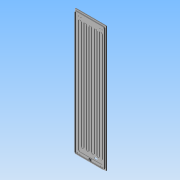
# Autodesk Inventor part: Ply back
Saved by Autodesk Inventor 2013 (Build 170138000, 138)
## iProperties
Created: 2018-07-07
Part Number: Ply back
Material: Generic
Document SubType Name: Modeling
Designer: Jeff Vyduna
Density: 1 g/cm^3
Author: Jeff Vyduna
Autodesk Inventor part; units mm, degrees
ref_plane "YZ Plane" through (0, 0, 0) normal (1, 0, 0) x (0, 1, 0)
ref_plane "XZ Plane" through (0, 0, 0) normal (0, 1, 0) x (-1, 0, 0)
ref_plane "XY Plane" through (0, 0, 0) normal (0, 0, 1) x (1, 0, 0)
sketch "TwoLineColumn" plane through (0, 0, 0) normal (0, 0, 1) x (1, 0, 0)
  line L0 (50.8, -1261.9609) -> (50.8, 922.4391) construction
  line L1 (101.6, -1261.9609) -> (101.6, 922.4391) construction
  arc A0 (101.6, 922.4391) -> (50.8, 922.4391) centre (76.2, 922.4391) ccw construction
  arc A1 (101.6, -1261.9609) -> (152.4, -1261.9609) centre (127, -1261.9609) ccw construction
  line L2 (56.896, -1261.9609) -> (56.896, 922.4391)
  arc A2 (95.504, 922.4391) -> (56.896, 922.4391) centre (76.2, 922.4391) ccw
  line L3 (95.504, 922.4391) -> (95.504, -1261.9609)
  arc A3 (95.504, -1261.9609) -> (158.496, -1261.9609) centre (127, -1261.9609) ccw
  line L4 (44.704, -1261.9609) -> (44.704, 922.4391)
  arc A4 (107.696, 922.4391) -> (44.704, 922.4391) centre (76.2, 922.4391) ccw
  line L5 (107.696, 922.4391) -> (107.696, -1261.9609)
  arc A5 (107.696, -1261.9609) -> (146.304, -1261.9609) centre (127, -1261.9609) ccw
  line L6 (50.8, -1261.9609) -> (152.4, -1261.9609) construction
  dimension "d4" = 2184.4
  dimension "lineSpacing" = 50.8
  dimension "d6" = 25.4
  dimension "d9" = 6.096
  dimension "d10" = 6.096
  measures "d4" distance of L0.start L0.end
  measures "lineSpacing" distance between parallel lines of L1 L0
  measures "d6" radius of A1
  measures "d9" distance between parallel lines of L1 L3
  measures "d10" distance between parallel lines of L5 L1
sketch "TwoLineColumnEnd" plane through (0, 0, 0) normal (0, 0, 1) x (1, 0, 0)
  line L0 (103.0524, -1453.1843) -> (103.0524, 731.2157)
  arc A0 (166.0444, 731.2157) -> (103.0524, 731.2157) centre (134.5484, 731.2157) ccw
  line L1 (166.0444, 731.2157) -> (166.0444, -1453.1843)
  line L2 (109.1484, -1453.1843) -> (109.1484, 731.2157) construction
  line L3 (159.9484, -1453.1843) -> (159.9484, 731.2157) construction
  arc A1 (159.9484, 731.2157) -> (109.1484, 731.2157) centre (134.5484, 731.2157) ccw construction
  line L4 (115.2444, -1453.1843) -> (115.2444, 731.2157)
  arc A2 (153.8524, 731.2157) -> (115.2444, 731.2157) centre (134.5484, 731.2157) ccw
  line L5 (153.8524, 731.2157) -> (153.8524, -1453.1843)
  line L6 (109.1484, -1453.1843) -> (159.9484, -1453.1843) construction
  dimension "d22" = 2184.4
  dimension "d23" = 50.8
  dimension "d25" = 6.096
  dimension "d26" = 6.096
  dimension "d29" = 50.8
  measures "d22" distance of L2.start L2.end
  measures "d23" distance between parallel lines of L3 L2
  measures "d25" distance between parallel lines of L3 L5
  measures "d26" distance between parallel lines of L1 L3
  measures "d29" distance of L2.start L6.end
sketch "15mm Neon profile" plane through (0, 0, 0) normal (0, 0, 1) x (1, 0, 0)
  circle A0 centre (522.6685, 24.7098) radius 6.985 construction
  line L0 (516.6995, 21.082) -> (528.6375, 21.082) construction
  line L1 (528.6375, 21.082) -> (528.6375, 6.35) construction
  line L2 (528.6375, 6.35) -> (516.6995, 6.35) construction
  line L3 (516.6995, 6.35) -> (516.6995, 21.082) construction
  point P0 (522.6685, 16.011)
  dimension "d73" = 13.97
  dimension "d74" = 11.938
  dimension "d76" = 14.732
  measures "d73" diameter of A0
  measures "d74" distance of L0.start L0.end
  measures "d76" distance of L0.end L1.end
sketch "U Bolt hole and bore" plane through (0, 0, 0) normal (0, 0, 1) x (1, 0, 0)
  circle A0 centre (40.0435, 30.4025) radius 9.525
  circle A1 centre (74.9685, 30.4025) radius 9.525
  circle A2 centre (40.0435, 30.4025) radius 3.9688
  circle A3 centre (74.9685, 30.4025) radius 3.9688
  point P0 (68.2625, 33.02)
  dimension "d100" = 19.05
  dimension "d102" = 34.925
  dimension "d105" = 7.9375
  measures "d100" diameter of A0
  measures "d102" distance of A1.centre A0.centre
  measures "d105" diameter of A2
sketch "Stock" plane through (0, 0, 0) normal (0, 0, 1) x (1, 0, 0)
  line L0 (0, 0) -> (604.8375, 0)
  line L1 (604.8375, 0) -> (604.8375, 2438.4)
  line L2 (604.8375, 2438.4) -> (0, 2438.4)
  line L3 (0, 2438.4) -> (0, 0)
  dimension "d1" = 604.8375
  dimension "d2" = 2438.4
  constraints: 8 end point, 2 parallel, 1 coincident, 1 horizontal, 1 perpendicular
  measures "d1" distance of L2.end L1.end
  measures "d2" distance of L1.end L0.end
extrude "Stock Extrusion" add sketch "Stock" along normal blind 19.05
sketch "LEDPocket" plane through (0, 0, 19.05) normal (0, 0, 1) x (1, 0, 0)
  line L0 (0, 0) -> (604.8375, 0)
  line L1 (604.8375, 0) -> (604.8375, 2438.4)
  line L2 (63.5, 2438.4) -> (63.5, 0) construction
  line L3 (541.3375, 2438.4) -> (541.3375, 0) construction
  line L4 (474.1228, 177.8) -> (474.1228, 2266.95)
  arc A0 (537.1148, 2266.95) -> (474.1228, 2266.95) centre (505.6188, 2266.95) ccw
  line L5 (537.1148, 2266.95) -> (537.1148, 88.9)
  line L6 (480.2188, 177.8) -> (480.2188, 2266.95) construction
  line L7 (531.0188, 177.8) -> (531.0188, 2266.95) construction
  arc A1 (531.0188, 2266.95) -> (480.2188, 2266.95) centre (505.6188, 2266.95) ccw construction
  line L8 (486.3148, 177.8) -> (486.3148, 2266.95)
  arc A2 (524.9228, 2266.95) -> (486.3148, 2266.95) centre (505.6188, 2266.95) ccw
  line L9 (524.9228, 2266.95) -> (524.9228, 152.4)
  line L10 (67.7227, 88.9) -> (67.7227, 2266.95)
  arc A3 (130.7147, 2266.95) -> (67.7227, 2266.95) centre (99.2187, 2266.95) ccw
  line L11 (130.7147, 2266.95) -> (130.7147, 177.8)
  arc A4 (130.7147, 177.8) -> (169.3227, 177.8) centre (150.0187, 177.8) ccw
  line L12 (73.8187, 177.8) -> (73.8187, 2266.95) construction
  line L13 (124.6187, 177.8) -> (124.6187, 2266.95) construction
  arc A5 (124.6187, 2266.95) -> (73.8187, 2266.95) centre (99.2187, 2266.95) ccw construction
  arc A6 (124.6187, 177.8) -> (175.4187, 177.8) centre (150.0187, 177.8) ccw construction
  line L14 (79.9147, 152.4) -> (79.9147, 2266.95)
  arc A7 (118.5227, 2266.95) -> (79.9147, 2266.95) centre (99.2187, 2266.95) ccw
  line L15 (118.5227, 2266.95) -> (118.5227, 177.8)
  arc A8 (118.5227, 177.8) -> (181.5147, 177.8) centre (150.0187, 177.8) ccw
  line L16 (169.3227, 177.8) -> (169.3227, 2266.95)
  arc A9 (232.3147, 2266.95) -> (169.3227, 2266.95) centre (200.8187, 2266.95) ccw
  line L17 (232.3147, 2266.95) -> (232.3147, 177.8)
  arc A10 (232.3147, 177.8) -> (270.9227, 177.8) centre (251.6187, 177.8) ccw
  line L18 (175.4187, 177.8) -> (175.4187, 2266.95) construction
  line L19 (226.2187, 177.8) -> (226.2187, 2266.95) construction
  arc A11 (226.2187, 2266.95) -> (175.4187, 2266.95) centre (200.8187, 2266.95) ccw construction
  arc A12 (226.2187, 177.8) -> (277.0187, 177.8) centre (251.6187, 177.8) ccw construction
  line L20 (181.5147, 177.8) -> (181.5147, 2266.95)
  arc A13 (220.1227, 2266.95) -> (181.5147, 2266.95) centre (200.8187, 2266.95) ccw
  line L21 (220.1227, 2266.95) -> (220.1227, 177.8)
  arc A14 (220.1227, 177.8) -> (283.1148, 177.8) centre (251.6187, 177.8) ccw
  line L22 (270.9227, 177.8) -> (270.9227, 2266.95)
  arc A15 (333.9147, 2266.95) -> (270.9227, 2266.95) centre (302.4187, 2266.95) ccw
  line L23 (333.9147, 2266.95) -> (333.9148, 177.8)
  arc A16 (333.9148, 177.8) -> (372.5227, 177.8) centre (353.2187, 177.8) ccw
  line L24 (277.0187, 177.8) -> (277.0187, 2266.95) construction
  line L25 (327.8187, 177.8) -> (327.8187, 2266.95) construction
  arc A17 (327.8187, 2266.95) -> (277.0187, 2266.95) centre (302.4187, 2266.95) ccw construction
  arc A18 (327.8187, 177.8) -> (378.6188, 177.8) centre (353.2187, 177.8) ccw construction
  line L26 (283.1148, 177.8) -> (283.1148, 2266.95)
  arc A19 (321.7227, 2266.95) -> (283.1148, 2266.95) centre (302.4187, 2266.95) ccw
  line L27 (321.7227, 2266.95) -> (321.7227, 177.8)
  arc A20 (321.7227, 177.8) -> (384.7148, 177.8) centre (353.2187, 177.8) ccw
  line L28 (372.5227, 177.8) -> (372.5227, 2266.95)
  arc A21 (435.5148, 2266.95) -> (372.5227, 2266.95) centre (404.0188, 2266.95) ccw
  line L29 (435.5148, 2266.95) -> (435.5148, 177.8)
  arc A22 (435.5148, 177.8) -> (474.1228, 177.8) centre (454.8188, 177.8) ccw
  line L30 (378.6188, 177.8) -> (378.6188, 2266.95) construction
  line L31 (429.4188, 177.8) -> (429.4188, 2266.95) construction
  arc A23 (429.4188, 2266.95) -> (378.6188, 2266.95) centre (404.0188, 2266.95) ccw construction
  arc A24 (429.4188, 177.8) -> (480.2188, 177.8) centre (454.8188, 177.8) ccw construction
  line L32 (384.7148, 177.8) -> (384.7148, 2266.95)
  arc A25 (423.3227, 2266.95) -> (384.7148, 2266.95) centre (404.0188, 2266.95) ccw
  line L33 (423.3227, 2266.95) -> (423.3227, 177.8)
  arc A26 (423.3227, 177.8) -> (486.3148, 177.8) centre (454.8188, 177.8) ccw
  line L34 (499.5228, 127) -> (105.3147, 127)
  line L35 (63.5, 2374.9) -> (541.3375, 2374.9) construction
  arc A27 (79.9147, 152.4) -> (105.3147, 127) centre (105.3147, 152.4) ccw
  arc A28 (67.7227, 88.9) -> (93.1227, 63.5) centre (93.1227, 88.9) ccw
  arc A29 (499.5228, 127) -> (524.9228, 152.4) centre (499.5228, 152.4) ccw
  arc A30 (511.7148, 63.5) -> (537.1148, 88.9) centre (511.7148, 88.9) ccw
  line L36 (93.1227, 63.5) -> (511.7148, 63.5)
  line L37 (0, 2438.4) -> (0, 0) projected
  line L38 (604.8375, 2438.4) -> (0, 2438.4) projected
  line L39 (63.5, 2311.4) -> (541.3375, 2311.4) construction
  point P0 (79.9147, 127)
  point P1 (524.9228, 127)
  dimension "d21" = 541.3375
  dimension "d42" = 50.8
  dimension "d43" = 6.096
  dimension "d44" = 6.096
  dimension "d50" = 50.8
  dimension "d51" = 25.4
  dimension "d52" = 6.096
  dimension "d53" = 6.096
  dimension "d202" = 50.8
  dimension "d204" = 25.4
  dimension "d205" = 63.5
  dimension "d206" = 63.5
  dimension "d208" = 302.4187
  dimension "d209" = 63.5
  dimension "d210" = 63.5
  dimension "d211" = 25.4
  dimension "d212" = 44.45
  dimension "d213" = 63.5
  constraints: 76 end point, 62 point on circle, 60 tangent, 31 centre point, 27 vertical, 12 point on line, 9 horizontal alignment, 8 equal radius, 2 horizontal, 1 perpendicular
  measures "d21" distance from line of L0.start L3
  measures "d42" distance between parallel lines of L7 L6
  measures "d43" distance between parallel lines of L7 L9
  measures "d44" distance between parallel lines of L5 L7
  measures "d50" distance between parallel lines of L13 L12
  measures "d51" radius of A6
  measures "d52" distance between parallel lines of L13 L15
  measures "d53" distance between parallel lines of L11 L13
  measures "d202" distance from line of L34 A4.centre
  measures "d204" radius of A27
  measures "d205" distance between parallel lines of L36 L34
  measures "d206" distance between parallel lines of L0 L36
  measures "d208" distance from line of L37 A15.centre
  measures "d209" distance from line of L35.start L38
  measures "d210" distance of L39.start L35.start
  measures "d211" radius of A28
  measures "d212" vertical distance of A3.centre L39.start
  measures "d213" distance from line of L0.start L2
extrude "Main rope pocket" cut sketch "LEDPocket" against normal blind 12.7 contours L4 A0 L5 A30 L36 A28 L10 A3 L11 A4 L16 A9 L17 A10 L22 A15 L23 A16 L28 A21 L29 A22
sketch "Side profile reference" plane through (0, 0, 0) normal (0, -1, 0) x (1, 0, 0)
  line L0 (0, 0) -> (604.8375, 0) projected
  line L1 (604.8375, 0) -> (604.8375, 19.05) projected
  line L2 (0, 19.05) -> (604.8375, 19.05) projected
  line L3 (0, 0) -> (0, 19.05) projected
  line L4 (598.4875, 38.1) -> (586.2955, 38.1) construction
  line L5 (586.2955, 38.1) -> (586.2955, 25.4) construction
  line L6 (586.2955, 25.4) -> (598.4875, 25.4) construction
  line L7 (598.4875, 25.4) -> (598.4875, 38.1) construction
  line L8 (604.8375, 19.05) -> (541.3375, 19.05) construction
  line L9 (541.3375, 19.05) -> (541.3375, 38.1) construction
  line L10 (541.3375, 38.1) -> (604.8375, 38.1) construction
  line L11 (604.8375, 38.1) -> (604.8375, 19.05) construction
  line L12 (547.6875, 38.1) -> (573.0875, 38.1) construction
  line L13 (573.0875, 38.1) -> (573.0875, 40.64) construction
  line L14 (573.0875, 40.64) -> (547.6875, 40.64) construction
  line L15 (547.6875, 40.64) -> (547.6875, 38.1) construction
  line L16 (579.4375, 40.64) -> (516.6995, 40.64) construction
  line L17 (516.6995, 40.64) -> (516.6995, 45.847) construction
  line L18 (516.6995, 45.847) -> (579.4375, 45.847) construction
  line L19 (579.4375, 45.847) -> (579.4375, 40.64) construction
  circle A0 centre (522.6685, 24.7098) radius 6.985 construction
  line L20 (516.6995, 21.082) -> (528.6375, 21.082) construction
  line L21 (528.6375, 21.082) -> (528.6375, 6.35) construction
  line L22 (528.6375, 6.35) -> (516.6995, 6.35) construction
  line L23 (516.6995, 6.35) -> (516.6995, 21.082) construction
  circle A1 centre (592.3915, 43.7598) radius 6.985 construction
  line L24 (586.4225, 40.132) -> (598.3605, 40.132) construction
  line L25 (598.3605, 40.132) -> (598.3605, 25.4) construction
  line L26 (598.3605, 25.4) -> (586.4225, 25.4) construction
  line L27 (586.4225, 25.4) -> (586.4225, 40.132) construction
  point P0 (566.7375, 19.05)
  point P1 (592.3915, 25.4)
  point P2 (592.3915, 25.4)
  dimension "d75" = 12.7
  dimension "d80" = 12.192
  dimension "d88" = 6.35
  dimension "d90" = 63.5
  dimension "d91" = 19.05
  dimension "d92" = 25.4
  dimension "d93" = 2.54
  dimension "d94" = 6.35
  dimension "d95" = 12.7
  dimension "d96" = 6.35
  dimension "d97" = 5.207
  dimension "d98" = 0
  dimension "d99" = 12.7
  constraints: 32 end point, 8 parallel, 5 horizontal, 4 perpendicular, 1 coincident, 1 collinear, 1 midpoint, 1 point on line, 1 other
  measures "d80" distance of L6.end L5.end
  measures "d88" horizontal distance of L1.end L6.end
  measures "d90" distance of L9.end L10.end
  measures "d91" distance of L8.end L9.end
  measures "d92" distance of L14.end L13.end
  measures "d93" distance of L13.end L12.end
  measures "d94" distance of L9.end L12.start
  measures "d96" horizontal distance of L16.start L12.end
  measures "d97" distance of L16.end L17.end
  measures "d99" vertical distance of L10.end L6.end
sketch "U-Bolt holes" plane through (0, 0, 19.05) normal (0, 0, 1) x (1, 0, 0)
  line L0 (0, 0) -> (604.8375, 0) projected
  line L1 (604.8375, 0) -> (604.8375, 2438.4) projected
  line L2 (0, 2438.4) -> (0, 0) projected
  line L3 (604.8375, 2438.4) -> (0, 2438.4) projected
  point P0 (53.975, 33.02)
  point P1 (100.0125, 33.02)
  point P2 (504.825, 33.02)
  point P3 (550.8625, 33.02)
  point P4 (531.8125, 2344.42)
  point P5 (485.775, 2344.42)
  point P6 (73.025, 2344.42)
  point P7 (119.0625, 2344.42)
  dimension "d109" = 33.02
  dimension "uBoltSpacing" = 46.0375
  dimension "d111" = 46.0375
  dimension "d112" = 19.05
  dimension "d113" = 53.975
  dimension "d114" = 53.975
  dimension "d115" = 46.0375
  dimension "d116" = 46.0375
  dimension "d117" = 19.05
  dimension "d126" = 93.98
  dimension "d198" = 2311.4
  constraints: 6 horizontal alignment
  measures "d109" distance from line of L0 point (53.975, 33.02)
  measures "uBoltSpacing" distance of point (100.012, 33.02) point (53.975, 33.02)
  measures "d111" distance of point (550.862, 33.02) point (504.825, 33.02)
  measures "d112" horizontal distance of point (53.975, 33.02) point (73.025, 2344.42)
  measures "d113" distance from line of L1 point (550.862, 33.02)
  measures "d114" distance from line of L2 point (53.975, 33.02)
  measures "d115" distance of point (73.025, 2344.42) point (119.062, 2344.42)
  measures "d116" distance of point (531.812, 2344.42) point (485.775, 2344.42)
  measures "d117" horizontal distance of point (531.812, 2344.42) point (550.862, 33.02)
  measures "d126" distance from line of L3 point (73.025, 2344.42)
  measures "d198" vertical distance of point (73.025, 2344.42) point (53.975, 33.02)
hole "Hole1" at (73.025, 2344.42, 19.05) at (119.0625, 2344.42, 19.05) at (485.775, 2344.42, 19.05) at (531.8125, 2344.42, 19.05) at (550.8625, 33.02, 19.05) at (504.825, 33.02, 19.05) at (100.0125, 33.02, 19.05) at (53.975, 33.02, 19.05) direction (0, 0, -1) diameter 7.9375 end through all counterbore diameter 19.05 counterbore depth 6.35
ref_plane "Work Plane1" through (0, 0, 6.35) normal (0, 0, 1) x (1, 0, 0)
sketch "WeatherProof panel" plane through (0, 0, 6.35) normal (0, 0, 1) x (1, 0, 0)
  line L0 (370.9353, 127) -> (418.5603, 127)
  line L1 (423.3228, 122.2375) -> (423.3228, 87.3125)
  line L2 (418.5603, 82.55) -> (370.9353, 82.55)
  line L3 (366.1728, 87.3125) -> (366.1728, 122.2375)
  arc A0 (370.9353, 127) -> (366.1728, 122.2375) centre (370.9353, 122.2375) ccw
  arc A1 (366.1728, 87.3125) -> (370.9353, 82.55) centre (370.9353, 87.3125) ccw
  arc A2 (423.3228, 122.2375) -> (418.5603, 127) centre (418.5603, 122.2375) ccw
  arc A3 (418.5603, 82.55) -> (423.3228, 87.3125) centre (418.5603, 87.3125) ccw
  line L4 (105.3147, 127) -> (499.5228, 127) projected
  line L5 (524.9228, 152.4) -> (524.9228, 2266.95) projected
  point P0 (0, 0)
  point P1 (423.3228, 82.55)
  point P2 (423.3228, 127)
  point P3 (366.1728, 82.55)
  dimension "d127" = 44.45
  dimension "d129" = 57.15
  dimension "d130" = 4.7625
  dimension "d214" = 101.6
  constraints: 8 end point, 8 point on circle, 8 tangent, 6 point on line, 4 centre point, 3 equal radius, 2 parallel, 1 collinear, 1 horizontal, 1 perpendicular
  measures "d127" distance of point (423.323, 127) point (423.323, 82.55)
  measures "d129" distance of point (423.323, 82.55) point (366.173, 82.55)
  measures "d130" radius of A0
  measures "d214" distance between parallel lines of L5 L1
extrude "Through Panel Extrusion5" cut sketch "WeatherProof panel" against normal through all
sketch "Border" plane through (0, 0, 19.05) normal (0, 0, 1) x (1, 0, 0)
  line L0 (38.989, 2418.461) -> (565.8485, 2418.461) construction
  line L1 (584.8985, 2399.411) -> (584.8985, 38.989) construction
  line L2 (19.939, 38.989) -> (19.939, 2399.411) construction
  line L3 (0, 2438.4) -> (0, 0) construction
  line L4 (604.8375, 2438.4) -> (0, 2438.4) construction
  line L5 (0, 0) -> (604.8375, 0) construction
  arc A0 (19.939, 38.989) -> (38.989, 19.939) centre (38.989, 38.989) ccw construction
  arc A1 (565.8485, 19.939) -> (584.8985, 38.989) centre (565.8485, 38.989) ccw construction
  arc A2 (584.8985, 2399.411) -> (565.8485, 2418.461) centre (565.8485, 2399.411) ccw construction
  arc A3 (38.989, 2418.461) -> (19.939, 2399.411) centre (38.989, 2399.411) ccw construction
  line L6 (511.7148, 63.5) -> (93.1227, 63.5) construction
  line L7 (315.1187, 63.5) -> (315.1187, 38.989) construction
  line L8 (289.7187, 38.989) -> (289.7187, 63.5) construction
  line L9 (565.8485, 19.939) -> (334.1687, 19.939) construction
  line L10 (270.6687, 19.939) -> (38.989, 19.939) construction
  arc A4 (270.6687, 19.939) -> (289.7187, 38.989) centre (270.6687, 38.989) ccw construction
  arc A5 (315.1187, 38.989) -> (334.1687, 19.939) centre (334.1687, 38.989) ccw construction
  line L11 (311.0547, 63.5) -> (311.0547, 38.989)
  arc A6 (311.0547, 38.989) -> (316.5711, 24.003) centre (334.1687, 38.989) ccw
  line L12 (38.989, 15.875) -> (565.8485, 15.875)
  arc A7 (565.8485, 15.875) -> (588.9625, 38.989) centre (565.8485, 38.989) ccw
  line L13 (588.9625, 38.989) -> (588.9625, 2399.411)
  arc A8 (588.9625, 2399.411) -> (565.8485, 2422.525) centre (565.8485, 2399.411) ccw
  line L14 (565.8485, 2422.525) -> (38.989, 2422.525)
  arc A9 (38.989, 2422.525) -> (15.875, 2399.411) centre (38.989, 2399.411) ccw
  line L15 (15.875, 2399.411) -> (15.875, 38.989)
  arc A10 (15.875, 38.989) -> (38.989, 15.875) centre (38.989, 38.989) ccw
  arc A11 (288.2664, 24.003) -> (293.7827, 38.989) centre (270.6687, 38.989) ccw
  line L16 (293.7827, 38.989) -> (293.7827, 63.5)
  line L17 (319.1827, 63.5) -> (319.1827, 38.989)
  arc A12 (319.1827, 38.989) -> (334.1687, 24.003) centre (334.1687, 38.989) ccw
  line L18 (334.1687, 24.003) -> (565.8485, 24.003)
  arc A13 (565.8485, 24.003) -> (580.8345, 38.989) centre (565.8485, 38.989) ccw
  line L19 (580.8345, 38.989) -> (580.8345, 2399.411)
  arc A14 (580.8345, 2399.411) -> (565.8485, 2414.397) centre (565.8485, 2399.411) ccw
  line L20 (565.8485, 2414.397) -> (38.989, 2414.397)
  arc A15 (38.989, 2414.397) -> (24.003, 2399.411) centre (38.989, 2399.411) ccw
  line L21 (24.003, 2399.411) -> (24.003, 38.989)
  arc A16 (24.003, 38.989) -> (38.989, 24.003) centre (38.989, 38.989) ccw
  line L22 (38.989, 24.003) -> (270.6687, 24.003)
  arc A17 (270.6687, 24.003) -> (285.6547, 38.989) centre (270.6687, 38.989) ccw
  line L23 (285.6547, 38.989) -> (285.6547, 63.5)
  arc A18 (293.7827, 63.5) -> (285.6547, 63.5) centre (289.7187, 63.5) ccw
  arc A19 (319.1827, 63.5) -> (311.0547, 63.5) centre (315.1187, 63.5) ccw
  line L24 (288.2664, 24.003) -> (316.5711, 24.003)
  line L25 (38.989, 15.875) -> (319.1827, 15.875)
  line L26 (334.1687, 15.875) -> (565.8485, 15.875)
  line L27 (604.8375, 0) -> (604.8375, 2438.4) projected
  point P0 (19.939, 2418.461)
  point P1 (584.8985, 2418.461)
  dimension "d227" = 19.05
  dimension "d228" = 19.939
  dimension "d229" = 19.05
  dimension "d230" = 25.4
  dimension "d231" = 8.128
  dimension "d232" = 4.064
  dimension "d233" = 8.128
  dimension "d234" = 8.128
  dimension "d235" = 8.128
  dimension "d240" = 19.939
  dimension "d241" = 19.939
  dimension "d242" = 19.939
  constraints: 46 end point, 41 point on circle, 22 tangent, 20 centre point, 13 parallel, 9 point on line, 4 equal radius, 4 perpendicular, 3 horizontal alignment, 1 collinear, 1 horizontal, 1 vertical, 18 other
  measures "d227" radius of A0
  measures "d228" distance between parallel lines of L5 L9
  measures "d229" radius of A4
  measures "d230" distance between parallel lines of L7 L8
  measures "d231" distance between parallel lines of L23 L16
  measures "d232" distance between parallel lines of L16 L8
  measures "d233" distance between parallel lines of L25 L24
  measures "d234" radial gap between concentric circles of A11 A17
  measures "d235" radial gap between concentric circles of A12 A6
  measures "d240" distance between parallel lines of L4 L0
  measures "d241" distance from line of L3.start L2
  measures "d242" distance from line of L27 L1.start
extrude "Outline Channel" add sketch "Border" along normal blind 25.4
equation "\"d4\" = litH"
equation "\"d6\" = 0.5 * lineSpacing"
equation "\"d9\" = 0.5 * pathW"
equation "\"d10\" = 0.5 * pathW"
equation "\"d22\" = litH"
equation "\"d25\" = 0.5 * pathW"
equation "\"d26\" = 0.5 * pathW"
equation "\"d29\" = lineSpacing"
equation "\"d1\" = signW"
equation "\"d2\" = signH"
equation "\"d21\" = signW - borderW"
equation "\"d51\" = 0.5 * d50"
equation "\"litH\" = 2184.4"
equation "\"borderW\" = 63.5"
equation "\"pathEndMillD\" = 9.525"
equation "\"signW\" = -0.5 * pathEndMillD + 0.5 * ply4x8w"
equation "\"pathW\" = 12.192"
equation "\"ply4x8w\" = 1219.2"
equation "\"signH\" = 2438.4"
equation "\"ePocketH\" = 63.5"
equation "\"minBendR\" = 25.4"
equation "\"outlineCOffset\" = 19.939"
equation "\"sRopeChannel\" = 8.128"
equation "\"sRopeDepth\" = 10.922"
equation "\"sRopeBendR\" = 19.05"
body "Solid1"
